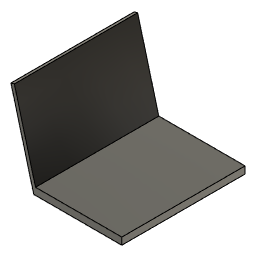
Laptop (Autodesk Fusion 360 design; units mm, degrees)
Autodesk Fusion 360 part; units mm, degrees
sketch "Schizzo1" plane through (0, 0, 0) normal (0, 1, 0) x (1, 0, 0)
  line L0 (0, 0) -> (-64.7048, -241.4815)
  line L1 (-64.7048, -241.4815) -> (-55.0455, -244.0696)
  line L2 (-55.0455, -244.0696) -> (4.9938, -20)
  line L3 (4.9938, -20) -> (250, -20)
  line L4 (250, -20) -> (250, 0)
  line L5 (250, 0) -> (0, 0)
  dimension "d1" = 75
  dimension "d2" = 250
  dimension "d3" = 250
  dimension "d4" = 20
  dimension "d5" = 10
  constraint coincident L0.start L5.end
  constraint perpendicular L0 L1
  constraint perpendicular L1 L2
  constraint horizontal L3
  constraint perpendicular L3 L4
  constraint horizontal L5
  measures "d1" angle of L0 L5
  measures "d2" distance of L0.start L4.end
  measures "d3" distance of L0.start L0.end
  measures "d4" distance of L3.end L4.end
  measures "d5" distance of L0.end L1.end
extrude "Estrusione1" add sketch "Schizzo1" along normal blind 350
component "Component" placed x (1, 0, 0) y (0, 1, 0) z (0, 0, 1) at (0, 0, 0)
